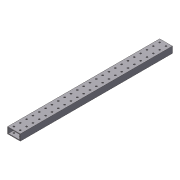
# Autodesk Inventor part: FrameCrossMember
Saved by Autodesk Inventor 2012 (Build 160160000, 160)
## iProperties
Created: 2013-01-08
Part Number: FrameCrossMember
Material: Aluminum-6061
Document SubType Name: Modeling
Designer: JesseK
Mass: 706.589 g
Surface Area: 1712.09 cm^2
Volume: 260.734 cm^3
Density: 2.71 g/cm^3
Author: JesseK
Autodesk Inventor part; units mm, degrees
ref_plane "YZ Plane" through (0, 0, 0) normal (1, 0, 0) x (0, 1, 0)
ref_plane "XZ Plane" through (0, 0, 0) normal (0, 1, 0) x (-1, 0, 0)
ref_plane "XY Plane" through (0, 0, 0) normal (0, 0, 1) x (1, 0, 0)
sketch "Sketch1" plane through (0, 0, 0) normal (0, 0, 1) x (1, 0, 0)
  line L0 (0, 0) -> (50.8, 0)
  line L1 (50.8, 0) -> (50.8, 25.4)
  line L2 (50.8, 25.4) -> (0, 25.4)
  line L3 (0, 25.4) -> (0, 0)
  dimension "d0" = 25.4
  dimension "d1" = 50.8
  constraints: 8 end point, 2 parallel, 1 horizontal, 1 perpendicular
  measures "d0" distance of L2.end L0.start
  measures "d1" distance of L1.end L2.end
extrude "Extrusion1" add sketch "Sketch1" along normal blind 609.6
shell "Shell1" thickness 3.175 removed faces 2 at (33.8667, 8.4667, 0) at (33.8667, 8.4667, 609.6)
sketch "Sketch2" plane through (0, 25.4, 0) normal (0, 1, 0) x (1, 0, 0)
  line L0 (50.8, 0) -> (0, 0) projected
  line L1 (0, 0) -> (0, -609.6) projected
  circle A0 centre (12.7, -12.7) radius 3.175
  dimension "d5" = 12.7
  dimension "d6" = 12.7
  dimension "d7" = 6.35
  constraints: 1 centre point
  measures "d5" distance from line of L1 A0.centre
  measures "d6" distance from line of L0 A0.centre
  measures "d7" diameter of A0
extrude "Extrusion2" cut sketch "Sketch2" against normal through all
pattern_linear "Rectangular Pattern1" count 24 spacing 25.4 along (0, 0, 1) count 2 spacing 25.4 along (1, 0, 0) of "Extrusion2"
body "Solid1"
